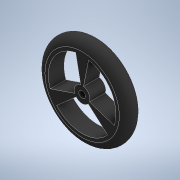
# Autodesk Inventor part: Wiel
Saved by Autodesk Inventor 2022 (Build 260153000, 153)
## iProperties
Created: 2022-10-15
Part Number: Wiel
Material: Rubber, Silicone
Document SubType Name: Modeling
Designer: gebruiker
Density: 1.25 g/cm^3
Appearance: Rubber - Black
Author: gebruiker
Autodesk Inventor part; units mm, degrees
ref_plane "YZ Plane" through (0, 0, 0) normal (1, 0, 0) x (0, 1, 0)
ref_plane "XZ Plane" through (0, 0, 0) normal (0, 1, 0) x (-1, 0, 0)
ref_plane "XY Plane" through (0, 0, 0) normal (0, 0, 1) x (1, 0, 0)
sketch "Sketch1" plane through (0, 0, 0) normal (0, 0, 1) x (1, 0, 0)
  circle A0 centre (0, 0) radius 20
  circle A1 centre (0, 0) radius 15
  dimension "d0" = 40
  dimension "d1" = 30
  constraints: 2 centre point, 2 coincident
  measures "d0" diameter of A0
  measures "d1" diameter of A1
extrude "Extrusion1" add sketch "Sketch1" along normal blind 7
fillet "Fillet1" radius 3.5 2 edges at (-20, 0, 7) (-20, 0, 0)
sketch "Sketch2" plane through (0, 0, 0) normal (0, 0, -1) x (-1, 0, 0)
  circle A0 centre (0, 0) radius 1.5
  circle A1 centre (0, 0) radius 3.5
  dimension "d5" = 3
  dimension "d6" = 7
  constraints: 2 centre point, 2 coincident
  measures "d5" diameter of A0
  measures "d6" diameter of A1
extrude "Extrusion2" add sketch "Sketch2" against normal blind 7
sketch "Sketch3" plane through (0, 0, 0) normal (0, 0, -1) x (-1, 0, 0)
  line L0 (-0.6265, 3.4435) -> (-2.8627, 14.7243)
  line L1 (-0.6265, 3.4435) -> (0.6262, 3.4435)
  line L2 (-0.6265, 3.4435) -> (0.6262, 3.4435) construction
  line L3 (0.6262, 3.4435) -> (2.8627, 14.7243)
  circle A0 centre (0, 0) radius 3.5
  circle A1 centre (0, 0) radius 15
  line L4 (-3.2952, -1.1794) -> (-14.183, -4.883)
  line L5 (-2.6689, -2.2643) -> (-11.3203, -9.8413)
  line L6 (2.669, -2.264) -> (11.3203, -9.8413)
  line L7 (3.2954, -1.1792) -> (14.183, -4.883)
  point P0 (2.6691, -2.2641)
  point P1 (0.6262, 3.4435)
  point P2 (-3.2953, -1.1795)
  dimension "d9" = 0
  dimension "d10" = 30
  dimension "d13" = 360
  constraints: 16 end point, 2 centre point, 2 coincident, 1 collinear, 1 horizontal, 19 other
  measures "d9" distance between parallel lines of L1 L2
  measures "d10" diameter of A1
extrude "Extrusion3" add sketch "Sketch3" against normal blind 7 contours L0 A1 L3 A0 | A0 L5 A1 L4 | L7 A1 L6 A0
body "Solid1"
